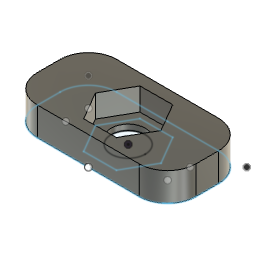
bracing for boat v1 (Autodesk Fusion 360 design; units mm, degrees)
Autodesk Fusion 360 part; units mm, degrees
sketch "Sketch1" plane through (0, 0, 0) normal (0, 0, 1) x (1, 0, 0)
  line L0 (2.861, 5.0148) -> (-2.9125, 4.9851)
  line L1 (-2.9125, 4.9851) -> (-5.7734, -0.0297)
  line L2 (-5.7734, -0.0297) -> (-2.861, -5.0148)
  line L3 (-2.861, -5.0148) -> (2.9125, -4.9851)
  line L4 (2.9125, -4.9851) -> (5.7734, 0.0297)
  line L5 (5.7734, 0.0297) -> (2.861, 5.0148)
  line L6 (-0.036, 6.9999) -> (-9.036, 6.9999)
  line L7 (-14.036, 1.9999) -> (-14.036, -2.0001)
  line L8 (-9.036, -7.0001) -> (-0.036, -7.0001)
  line L9 (-0.036, 6.9999) -> (8.964, 6.9999)
  line L10 (13.964, 1.9999) -> (13.964, -2.0001)
  line L11 (8.964, -7.0001) -> (-0.036, -7.0001)
  arc A0 (-9.036, 6.9999) -> (-14.036, 1.9999) centre (-9.036, 1.9999) ccw
  arc A1 (-14.036, -2.0001) -> (-9.036, -7.0001) centre (-9.036, -2.0001) ccw
  arc A2 (13.964, 1.9999) -> (8.964, 6.9999) centre (8.964, 1.9999) ccw
  arc A3 (8.964, -7.0001) -> (13.964, -2.0001) centre (8.964, -2.0001) ccw
  circle A4 centre (0, 0) radius 3
  point P0 (-14.036, 6.9999)
  point P1 (13.964, 6.9999)
  dimension "d1" = 5
  dimension "d3" = 14
  dimension "d4" = 14
  dimension "d5" = 14
  dimension "d6" = 14
  dimension "d7" = 5
  dimension "d8" = 5
  dimension "d9" = 5
  dimension "d10" = 5
  dimension "d11" = 6
  constraint coincident A4.centre origin
  constraint horizontal L6
  constraint vertical L7
  constraint horizontal L8
  constraint horizontal L9
  constraint vertical L10
  constraint horizontal L11
  constraint coincident P0 L7
  constraint coincident P0 L6
  constraint tangent L7 A0
  constraint tangent L6 A0
  constraint tangent L7 A1
  constraint tangent L8 A1
  constraint coincident P1 L9
  constraint coincident P1 L10
  constraint tangent L9 A2
  constraint tangent L10 A2
  constraint tangent L11 A3
  constraint tangent L10 A3
  measures "d1" distance of A4.centre L5
  measures "d3" distance of L6.start P0
  measures "d4" distance of L6.start L8.end
  measures "d5" distance of L6.start P1
  measures "d6" distance of L6.start L8.end
  measures "d7" radius of A0
  measures "d8" radius of A1
  measures "d9" radius of A2
  measures "d10" radius of A3
  measures "d11" diameter of A4
extrude "Extrude1" add sketch "Sketch1" along normal blind 5 contours L6 L7 L8 L9 L10 L11 A0 A1 A2 A3
extrude "Extrude2" add sketch "Sketch1" along normal blind 1 contours L0 L1 L2 L3 L4 L5
